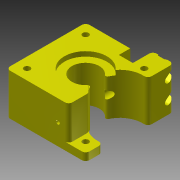
# Autodesk Inventor part: block
Saved by Autodesk Inventor 2013 (Build 170138000, 138)
## iProperties
Created: 2013-12-21
Part Number: block
Material: Generic
Document SubType Name: Modeling
Designer: employee
Density: 1 g/cm^3
Mass: 26.273 g
Surface Area: 85.4271 cm^2
Volume: 26.273 cm^3
Author: employee
Autodesk Inventor part; units mm, degrees
ref_plane "YZ Plane" through (0, 0, 0) normal (1, 0, 0) x (0, 1, 0)
ref_plane "XZ Plane" through (0, 0, 0) normal (0, 1, 0) x (-1, 0, 0)
ref_plane "XY Plane" through (0, 0, 0) normal (0, 0, 1) x (1, 0, 0)
sketch "Sketch1" plane through (0, 0, 0) normal (0, 0, 1) x (1, 0, 0)
  line L0 (-21, 21) -> (21, 21)
  line L1 (21, 21) -> (21, -21)
  line L2 (21, -21) -> (-21, -21)
  line L3 (-21, -21) -> (-21, 21)
  point P0 (0, 0)
  point P1 (-21, 0)
  point P2 (0, 21)
  dimension "d0" = 42
  constraints: 8 end point, 2 midpoint, 2 parallel, 2 perpendicular, 1 horizontal, 1 horizontal alignment, 1 vertical alignment
  measures "d0" distance of L2.end L0.start
extrude "Extrusion1" add sketch "Sketch1" along normal mid plane 22
sketch "Sketch3" plane through (0, 0, 11) normal (0, 0, 1) x (1, 0, 0)
  circle A0 centre (0, 0) radius 7.25
  dimension "d4" = 14.5
  constraints: 1 centre point, 1 coincident
  measures "d4" diameter of A0
extrude "Extrusion2" cut sketch "Sketch3" against normal through all
sketch "Sketch4" plane through (0, 0, 11) normal (0, 0, 1) x (1, 0, 0)
  circle A0 centre (0, 0) radius 7.25 projected
  line L0 (21, -21) -> (21, 21) projected
  circle A1 centre (0, 0) radius 5.3975
  circle A2 centre (18.1475, 0) radius 11
  line L1 (0, 0) -> (5.3975, 0)
  line L2 (5.3975, 0) -> (7.1475, 0)
  circle A3 centre (18.1475, 0) radius 12
  dimension "d9" = 10.795
  dimension "d12" = 22
  dimension "d11" = 1.75
  dimension "d14" = 24
  constraints: 4 end point, 3 horizontal alignment, 2 coincident, 1 centre point, 1 collinear, 1 perpendicular, 4 other
  measures "d11" distance of L1.end L2.end
  measures "d14" diameter of A3
extrude "Extrusion3" cut sketch "Sketch4" against normal through all contours A0 A2 | A0 A2 L0 | A2 L2 A3 A0 | A0 A3 L0 A2 | A2 L0 A3 A0 | A0 A3 L2 A2 | A2 L0 | L0 A3 A2
sketch "Sketch5" plane through (-21, -21, -11) normal (0, -1, 0) x (1, 0, 0)
  line L0 (42, 0) -> (0, 0) projected
  line L1 (0, 22) -> (42, 22) projected
  line L2 (15.6025, 22) -> (26.3975, 22)
  line L3 (26.3975, 22) -> (26.3975, 0)
  line L4 (26.3975, 0) -> (15.6025, 0)
  line L5 (15.6025, 0) -> (15.6025, 22)
  circle A0 centre (27.2725, 11) radius 0.875
  circle A1 centre (27.2725, 11) radius 1
  point P0 (21, 11)
  point P1 (21, 0)
  point P2 (21, 22)
  point P3 (26.3975, 11)
  dimension "d18" = 10.795
  dimension "d20" = 1.75
  dimension "d21" = 2
  constraints: 8 end point, 4 midpoint, 2 centre point, 2 parallel, 1 coincident, 1 horizontal, 1 horizontal alignment, 1 perpendicular, 1 tangent, 2 other
  measures "d18" distance between parallel lines of L3 L5
  measures "d20" diameter of A0
  measures "d21" diameter of A1
extrude "Extrusion4" cut sketch "Sketch5" against normal through all contours A1 L3 | A0 | L3 A1
sketch "Sketch6" plane through (-21, 21, -11) normal (0, 1, 0) x (1, 0, 0)
  circle A0 centre (27.2725, -11) radius 1 projected
  circle A1 centre (27.2725, -11) radius 2.1
  point P0 (21, -11)
  dimension "d24" = 4.2
  constraints: 1 centre point, 1 coincident
  measures "d24" diameter of A1
extrude "Extrusion5" cut sketch "Sketch6" against normal up to next
sketch "Sketch7" plane through (0, 0, 11) normal (0, 0, 1) x (1, 0, 0)
  arc A0 (6.5545, 3.0986) -> (6.5545, -3.0986) centre (0, 0) ccw projected
  line L0 (-15.5, 15.5) -> (15.5, 15.5) construction
  line L1 (15.5, 15.5) -> (15.5, -15.5) construction
  line L2 (15.5, -15.5) -> (-15.5, -15.5) construction
  line L3 (-15.5, -15.5) -> (-15.5, 15.5) construction
  circle A1 centre (-15.5, 15.5) radius 1.6
  circle A2 centre (15.5, 15.5) radius 1.6
  circle A3 centre (15.5, -15.5) radius 1.6
  circle A4 centre (-15.5, -15.5) radius 1.6
  point P0 (4.593, -5.2825)
  point P1 (4.593, 5.2825)
  dimension "d28" = 31
  dimension "d29" = 3.2
  constraints: 8 end point, 5 coincident, 4 centre point, 3 equal radius, 1 horizontal, 10 other
  measures "d28" distance of L0.start L0.end
  measures "d29" diameter of A4
extrude "Extrusion6" cut sketch "Sketch7" against normal through all
sketch "Sketch8" plane through (0, 0, 11) normal (0, 0, 1) x (1, 0, 0)
  arc A0 (6.5545, 3.0986) -> (6.5545, -3.0986) centre (0, 0) ccw projected
  circle A1 centre (0, 0) radius 11.25
  point P0 (4.593, -5.2825)
  point P1 (4.593, 5.2825)
  dimension "d32" = 22.5
  constraints: 1 centre point, 1 coincident, 1 other
  measures "d32" diameter of A1
extrude "Extrusion7" cut sketch "Sketch8" against normal blind 2.5
sketch "Sketch11" plane through (-21, 21, -11) normal (0, 1, 0) x (1, 0, 0)
  circle A0 centre (27.2725, -11) radius 2.1 projected
  line L0 (42, -22) -> (0, -22) projected
  line L1 (25.1725, -11) -> (25.1725, -22)
  line L2 (29.3725, -11) -> (29.3725, -22)
  point P0 (21, -11)
  constraints: 4 end point, 2 perpendicular, 2 point on circle, 2 point on line, 2 tangent
extrude "Extrusion10" cut sketch "Sketch11" against normal blind 2.5 contours L2 L0 L1 A0
sketch "Sketch12" plane through (-21, 18.5, -11) normal (0, 1, 0) x (1, 0, 0)
  line L0 (25.1725, -22) -> (25.1725, -11) projected
  line L1 (29.3725, -22) -> (25.1725, -22) projected
  line L2 (29.3725, -11) -> (29.3725, -22) projected
  arc A0 (25.1725, -11) -> (29.3725, -11) centre (27.2725, -11) ccw projected
  line L3 (27.2725, -6.7276) -> (30.9725, -8.8638)
  line L4 (30.9725, -8.8638) -> (30.9725, -13.1362)
  line L5 (30.9725, -13.1362) -> (27.2725, -15.2724)
  line L6 (27.2725, -15.2724) -> (23.5725, -13.1362)
  line L7 (23.5725, -13.1362) -> (23.5725, -8.8638)
  line L8 (23.5725, -8.8638) -> (27.2725, -6.7276)
  line L9 (23.5725, -13.1362) -> (23.5725, -22)
  line L10 (23.5725, -22) -> (25.1725, -22)
  line L11 (29.3725, -22) -> (30.9725, -22)
  line L12 (30.9725, -22) -> (30.9725, -13.1362)
  point P0 (21, -11)
  dimension "d44" = 7.4
  constraints: 20 end point, 2 collinear, 2 perpendicular, 1 coincident, 1 vertical, 13 other
  measures "d44" distance between parallel lines of L4 L7
extrude "Extrusion11" cut sketch "Sketch12" against normal blind 3.5
sketch "Sketch13" plane through (-21, 21, -11) normal (0, 1, 0) x (1, 0, 0)
  line L0 (42, -22) -> (29.3725, -22) projected
  line L1 (25.1725, -22) -> (0, -22) projected
  line L2 (25.1725, -22) -> (29.3725, -22)
  line L3 (27.2725, -22) -> (23.5725, -19.8638)
  line L4 (23.5725, -19.8638) -> (23.5725, -15.5914)
  line L5 (23.5725, -15.5914) -> (27.2725, -13.4552)
  line L6 (27.2725, -13.4552) -> (30.9725, -15.5914)
  line L7 (30.9725, -15.5914) -> (30.9725, -19.8638)
  line L8 (30.9725, -19.8638) -> (27.2725, -22)
  line L9 (23.5725, -19.8638) -> (23.5725, -22)
  line L10 (23.5725, -22) -> (25.1725, -22)
  line L11 (29.3725, -22) -> (30.9725, -22)
  line L12 (30.9725, -19.8638) -> (30.9725, -22)
  line L13 (23.5725, -22) -> (27.2725, -22)
  line L14 (27.2725, -22) -> (30.9725, -22)
  point P0 (21, -11)
  point P1 (27.2725, -17.7276)
  dimension "d48" = 7.4
  constraints: 26 end point, 3 collinear, 3 perpendicular, 2 point on line, 1 midpoint, 1 vertical, 13 other
  measures "d48" distance between parallel lines of L4 L7
extrude "Extrusion12" cut sketch "Sketch13" against normal up to surface (6 mm away)
sketch "Sketch22" plane through (21, -21, 11) normal (1, 0, 0) x (0, 0, -1)
  line L0 (0, 0) -> (22, 0) projected
  line L1 (4, 0) -> (18, 0)
  line L2 (18, 0) -> (18, 21)
  line L3 (18, 21) -> (4, 21)
  line L4 (4, 21) -> (4, 0)
  line L5 (0, 0) -> (4, 0)
  line L6 (4, 0) -> (4, 21)
  line L7 (4, 21) -> (0, 21)
  line L8 (0, 21) -> (0, 0)
  point P0 (11, 21)
  point P1 (11, 0)
  point P2 (11, 21)
  dimension "d76" = 14
  constraints: 16 end point, 4 parallel, 3 midpoint, 2 horizontal, 2 perpendicular, 1 coincident, 1 point on line
  measures "d76" distance of L2.end L3.end
extrude "Extrusion20" cut sketch "Sketch22" against normal blind 9
sketch "Sketch23" plane through (21, 21, 11) normal (1, 0, 0) x (0, 0, -1)
  line L0 (0, -9.344) -> (22, -9.344) projected
  line L1 (22, 0) -> (22, -9.344) projected
  line L2 (0, 0) -> (22, 0) projected
  line L3 (0, -9.344) -> (0, 0) projected
  line L4 (1.3736, 4.6) -> (4.7539, 0.5715)
  arc A0 (4.7539, 0.5715) -> (7.2053, 2.6285) centre (5.9796, 1.6) ccw
  line L5 (7.2053, 2.6285) -> (5.5509, 4.6)
  line L6 (5.5509, 4.6) -> (11.3736, 4.6)
  line L7 (11.3736, 4.6) -> (14.7539, 0.5715)
  arc A1 (14.7539, 0.5715) -> (17.2053, 2.6285) centre (15.9796, 1.6) ccw
  line L8 (17.2053, 2.6285) -> (15.5509, 4.6)
  line L9 (15.5509, 4.6) -> (22, 4.6)
  line L10 (22, 4.6) -> (22, 0)
  line L11 (1.3736, 4.6) -> (0, 4.6)
  line L12 (0, 4.6) -> (0, 0)
  line L13 (15.9796, 1.6) -> (22, 1.6) construction
  line L14 (5.9796, 1.6) -> (0, 2.3) construction
  point P0 (11, -21)
  dimension "d80" = 10
  dimension "d82" = 1.6
  dimension "d83" = 3
  dimension "d84" = 130
  constraints: 22 end point, 6 tangent, 5 parallel, 4 point on circle, 3 perpendicular, 2 centre point, 2 horizontal alignment, 1 equal length, 1 equal radius, 1 midpoint, 1 point on line, 1 vertical
  measures "d80" distance of L13.start L14.start
  measures "d82" radius of A1
  measures "d83" distance between parallel lines of L9 L13
  measures "d84" angle of L13 L8
extrude "Extrusion21" add sketch "Sketch23" against normal blind 5 contours L12 L11 L4 A0 L2 | L2 A1 L8 L9 L10 | A0 L5 L6 L7 A1 L2
sketch "Sketch24" plane through (16, 21, 11) normal (-1, 0, 0) x (0, 0, 1)
  line L0 (-5.9796, 0) -> (-15.9796, 0) projected
  arc A0 (-7.2053, 2.6285) -> (-5.9796, 0) centre (-5.9796, 1.6) ccw projected
  line L1 (-7.2053, 2.6285) -> (-5.5509, 4.6) projected
  line L2 (-5.5509, 4.6) -> (-11.3736, 4.6) projected
  line L3 (-11.3736, 4.6) -> (-14.7539, 0.5715) projected
  arc A1 (-15.9796, 0) -> (-14.7539, 0.5715) centre (-15.9796, 1.6) ccw projected
  line L4 (0, 0) -> (-5.9796, 0) projected
  line L5 (0, 0) -> (0, 4.6) projected
  line L6 (0, 4.6) -> (-1.3736, 4.6) projected
  line L7 (-1.3736, 4.6) -> (-4.7539, 0.5715) projected
  arc A2 (-5.9796, 0) -> (-4.7539, 0.5715) centre (-5.9796, 1.6) ccw projected
  line L8 (-22, 4.6) -> (0, 4.6)
  line L9 (0, 4.6) -> (0, 0)
  line L10 (0, 0) -> (-22, 0)
  line L11 (-22, 0) -> (-22, 4.6)
  point P0 (-11, -21)
  constraints: 8 end point, 2 parallel, 1 horizontal, 1 perpendicular
extrude "Extrusion22" add sketch "Sketch24" along normal up to surface (6.0275 mm away)
sketch "Sketch25" plane through (16, 21, 11) normal (1, 0, 0) x (0, 0, -1)
  line L0 (1.3736, 4.6) -> (4.7539, 0.5715) projected
  arc A0 (4.7539, 0.5715) -> (7.2053, 2.6285) centre (5.9796, 1.6) ccw projected
  line L1 (7.2053, 2.6285) -> (5.5509, 4.6) projected
  line L2 (1.3736, 4.6) -> (5.5509, 4.6) construction
  line L3 (17.2053, 2.6285) -> (15.5509, 4.6) projected
  line L4 (11.3736, 4.6) -> (15.5509, 4.6) construction
  line L5 (11.3736, 4.6) -> (14.7539, 0.5715) projected
  arc A1 (14.7539, 0.5715) -> (17.2053, 2.6285) centre (15.9796, 1.6) ccw projected
  line L6 (16.2038, 6) -> (18.2777, 3.5284)
  arc A2 (13.6815, -0.3284) -> (18.2777, 3.5284) centre (15.9796, 1.6) ccw
  line L7 (13.6815, -0.3284) -> (8.3713, 6)
  line L8 (8.3713, 6) -> (16.2038, 6)
  line L9 (6.2038, 6) -> (8.2777, 3.5284)
  arc A3 (3.6815, -0.3284) -> (8.2777, 3.5284) centre (5.9796, 1.6) ccw
  line L10 (3.6815, -0.3284) -> (-1.6287, 6)
  line L11 (-1.6287, 6) -> (6.2038, 6)
  point P0 (11, -21)
  dimension "d89" = 3
  constraints: 12 end point, 4 point on circle, 2 centre point, 1 equal radius, 6 other
  measures "d89" radius of A3
extrude "Extrusion23" cut sketch "Sketch25" against normal blind 3
fillet "Fillet5" radius 2 16 edges at (9.9725, 25.6, 0) (9.9725, 21, -3.2043) (-21, 21, 0) (-21, -21, 0) (21, 25.6, 10.3132) (16, 25.6, 10.3132) (21, 25.6, 2.5377) (16, 25.6, 4.5353) (16, 25.6, 0.5402) (16, 25.6, -5.4647) (21, 25.6, -7.7755) (21, 11.656, 0) (21, -11.656, -9) (21, -21, -9) (12, -21, 2) (12, -10.3057, 2)
fillet "Fillet6" radius 1 4 edges at (6.5545, 3.0986, -6.5405) (6.5545, 3.0986, 5.2905) (6.5545, -3.0986, 4.7297) (6.5545, -3.0986, -5.9797)
sketch "Sketch18" plane through (21, 21, 11) normal (1, 0, 0) x (0, 0, -1)
  line L0 (0, -9.344) -> (0, 0) projected
  line L1 (0, -3.9) -> (22, -3.9) projected
  circle A0 centre (4, -2.3) radius 1.6
  circle A1 centre (12, -2.3) radius 1.6
  point P0 (11, -21)
  dimension "d62" = 4
  dimension "d63" = 12
  dimension "d64" = 3.2
  constraints: 2 centre point, 2 tangent, 1 equal radius
  measures "d62" distance from line of A0.centre L0
  measures "d63" distance from line of A1.centre L0
  measures "d64" diameter of A0
sketch "Sketch19" plane through (21, 21, 11) normal (1, 0, 0) x (0, 0, -1)
  circle A0 centre (4, -2.3) radius 1.6 projected
  circle A1 centre (12, -2.3) radius 1.6 projected
  line L0 (0, 0) -> (22, 0) projected
  line L1 (2.4, -2.3) -> (2.4, 0)
  line L2 (5.6, -2.3) -> (5.6, 0)
  line L3 (10.4, -2.3) -> (10.4, 0)
  line L4 (13.6, -2.3) -> (13.6, 0)
  point P0 (11, -21)
  constraints: 8 end point, 4 point on circle, 4 point on line, 4 tangent, 3 perpendicular, 1 parallel
sketch "Sketch20" plane through (13.9, 21, 10) normal (1, 0, 0) x (0, 0, -1)
  arc A0 (10.4, -2.3) -> (13.6, -2.3) centre (12, -2.3) ccw projected
  arc A1 (2.4, -2.3) -> (5.6, -2.3) centre (4, -2.3) ccw projected
  line L0 (5.6, 0) -> (5.6, -2.3) projected
  line L1 (2.4, 0) -> (5.6, 0) projected
  line L2 (2.4, -2.3) -> (2.4, 0) projected
  circle A2 centre (4, -2.3) radius 3
  circle A3 centre (12, -2.3) radius 3
  point P0 (10, -21)
  dimension "d69" = 6
  constraints: 2 centre point, 2 coincident, 1 equal radius
  measures "d69" diameter of A3
sketch "Sketch21" plane through (10.9, 21, 10) normal (1, 0, 0) x (0, 0, -1)
  line L0 (2.0739, 0) -> (5.9261, 0) projected
  arc A0 (2.0739, 0) -> (5.9261, 0) centre (4, -2.3) ccw projected
  line L1 (10.0739, 0) -> (13.9261, 0) projected
  arc A1 (10.0739, 0) -> (13.9261, 0) centre (12, -2.3) ccw projected
  line L2 (1, -2.3) -> (1, 0)
  line L3 (1, 0) -> (2.0739, 0)
  line L4 (7, -2.3) -> (7, 0)
  line L5 (7, 0) -> (5.9261, 0)
  line L6 (9, -2.3) -> (9, 0)
  line L7 (9, 0) -> (10.0739, 0)
  line L8 (15, -2.3) -> (15, 0)
  line L9 (15, 0) -> (13.9261, 0)
  point P0 (10, -21)
  constraints: 16 end point, 7 perpendicular, 4 point on circle, 4 tangent, 1 horizontal
body "Solid1"
